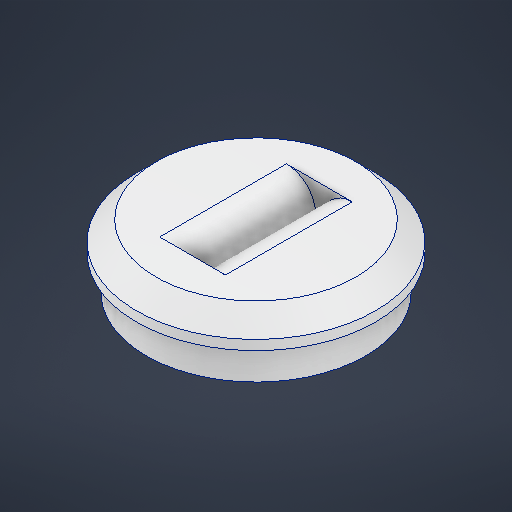
# Autodesk Inventor part: head_innter_top
Saved by Autodesk Inventor 2026.1 (Build 301233000, 233)
## iProperties
Created: 2026-04-17
Part Number: head_innter_top
Material: Aluminum 6061
Document SubType Name: Modeling
Designer: aaron
Density: 2.7 g/cm^3
Appearance: Aluminum - Flat
Author: aaron
Autodesk Inventor part; units mm, degrees
ref_plane "YZ Plane" through (0, 0, 0) normal (1, 0, 0) x (0, 1, 0)
ref_plane "XZ Plane" through (0, 0, 0) normal (0, 1, 0) x (-1, 0, 0)
ref_plane "XY Plane" through (0, 0, 0) normal (0, 0, 1) x (1, 0, 0)
sketch "Sketch1" plane through (0, 0, 0) normal (0, 0, 1) x (1, 0, 0)
  line L0 (0, 0) -> (0, 13)
  line L1 (0, 13) -> (22.5, 13)
  line L2 (22.5, 13) -> (24.5, 13)
  line L3 (24.5, 13) -> (24.5, 7)
  line L4 (24.5, 7) -> (22.5, 7)
  line L5 (22.5, 7) -> (22.5, 0)
  line L6 (22.5, 0) -> (0, 0)
  dimension "d0" = 13
  dimension "d3" = 22.5
  dimension "d4" = 2
  dimension "d5" = 6
  dimension "d6" = 2
  dimension "d7" = 7
  constraints: 14 end point, 3 perpendicular, 1 horizontal, 1 point on line, 1 vertical
  measures "d0" distance of L0.start L0.end
  measures "d3" distance of L0.end L1.end
  measures "d4" distance of L1.end L2.end
  measures "d5" distance of L2.end L3.end
  measures "d6" distance of L3.end L4.end
  measures "d7" distance of L4.end L5.end
revolve "Revolution1" add sketch "Sketch1" angle 360 about axis through (0, 0, 0) along (0, 1, 0)
sketch "Sketch2" plane through (0, 13, 0) normal (0, 1, 0) x (1, 0, 0)
  line L0 (0.75, 13) -> (-0.75, 13)
  line L1 (-0.75, 13) -> (-0.75, -13)
  line L2 (-0.75, -13) -> (0.75, -13)
  line L3 (0.75, -13) -> (0.75, 13)
  point P0 (0, 0)
  dimension "d9" = 1.5
  dimension "d10" = 26
  dimension "d11" = 13
  dimension "d12" = 0.75
  constraints: 8 end point, 2 parallel, 1 horizontal, 1 perpendicular
  measures "d9" distance between parallel lines of L3 L1
  measures "d10" distance of L2.end L0.start
  measures "d11" distance from line of point (0, 0) L2
  measures "d12" distance from line of L1 point (0, 0)
extrude "Extrusion1" cut sketch "Sketch2" against normal through all
fillet "Fillet1" radius 6 4 edges at (-0.75, 13, 0) (0.75, 13, 0) (-0.75, 0, 0) (0.75, 0, 0)
chamfer "Chamfer1" distance 4 angle 45 1 edges at (-24.5, 13, 0)
equation "\"d11\" = 0.5 * d10"
equation "\"d12\" = 0.5 * d9"
body "Solid1"
